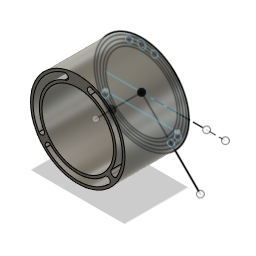
dc-15s_speaker_assembly (Autodesk Fusion 360 design; units mm, degrees)
Autodesk Fusion 360 part; units mm, degrees
sketch "Sketch1" plane through (0, 0, 0) normal (0, 0, 1) x (1, 0, 0)
  circle A0 centre (0, 0) radius 18.5
  circle A1 centre (0, 0) radius 14.05
  line L0 (-14.05, 0) -> (14.05, 0)
  line L1 (-14.05, -6.5) -> (14.05, -6.5)
  circle A2 centre (0, 0) radius 16.25
  line L2 (0, 0) -> (-18.0063, -18.0063)
  line L3 (0, 0) -> (25.4648, 0) construction
  line L4 (0, 0) -> (23.019, -23.019)
  line L5 (0, 0) -> (32.8468, 0) construction
  circle A3 centre (-11.4905, -11.4905) radius 1.25
  circle A4 centre (11.5095, -11.5095) radius 1.25
  circle A5 centre (0, 0) radius 17.5
  circle A6 centre (0, 0) radius 15.05
  circle A7 centre (0, 16.25) radius 1.55
  circle A8 centre (-4.9439, 15.4797) radius 1.275
  circle A9 centre (5.0183, 15.4557) radius 1.275
  circle A10 centre (-14.2746, -7.7652) radius 1.275
  circle A11 centre (14.2045, -7.8926) radius 1.275
  dimension "d1" = 37
  dimension "d2" = 28.1
  dimension "d3" = 6.5
  dimension "d11" = -2.25
  dimension "d12" = 135
  dimension "d13" = 45
  dimension "d14" = 2.5
  dimension "d15" = 2.5
  dimension "d16" = -1
  dimension "d17" = 1
  dimension "d18" = 3.1
  dimension "d19" = 2.55
  dimension "d20" = 2.55
  dimension "d21" = 2.55
  dimension "d22" = 2.55
  constraint coincident A0.centre A1.centre
  constraint concentric A0 A1
  constraint coincident A1 L0.start
  constraint coincident A1 L0.end
  constraint horizontal L0
  constraint horizontal L3
  constraint horizontal L5
  constraint coincident A2 A3.centre
  constraint coincident L2 A3.centre
  constraint midpoint L4 A4.centre
  constraint coincident A2 A7.centre
  constraint coincident A2 A8.centre
  constraint coincident A2 A9.centre
  constraint coincident A2 A10.centre
  constraint coincident A2 A11.centre
  measures "d1" diameter of A0
  measures "d2" diameter of A1
  measures "d12" angle of L2 L3
  measures "d13" angle of L4 L5
  measures "d14" diameter of A3
  measures "d15" diameter of A4
  measures "d18" diameter of A7
  measures "d19" diameter of A8
  measures "d20" diameter of A9
  measures "d21" diameter of A10
  measures "d22" diameter of A11
extrude "Extrude2" add sketch "Sketch1" along normal blind 1.5 contours A1 L0 L1 L2 | L1 L2 L4 | A1 L0 | A1 L0 L1 L4
extrude "Extrude1" add sketch "Sketch1" along normal blind 25 contours A0 L2 L4 A4 A5 A7 A8 A9 A10 A11 | A0 L2 L4 A4 A5 | A2 A3 A5 A10 | A2 A3 A6 A10 | A5 A10 | A2 A4 A5 A11 | A1 L1 L2 A3 A6 A10 | A1 L2 L4 A3 A4 A6 | A5 A8 | A2 A4 A6 A11 | A1 L1 L4 A4 A6 A11 | A2 A5 A7 A8 | A1 L1 A6 A7 A8 A9 | A2 A6 A7 A8 | A5 A7 | A2 A5 A7 | A5 A9 | A2 A6 A7 | A2 A5 A7 A9 | A2 A6 A7 A9 | A6 A7
